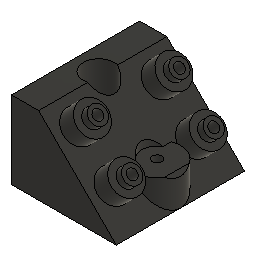
camera_block_left (Autodesk Fusion 360 design; units mm, degrees)
Autodesk Fusion 360 part; units mm, degrees
note: some values were not read from the file. Chosen so that the rebuilt part matches the saved one: which bodies a step acts on.
sketch "Skizze1" plane through (0, 0, 0) normal (0, 0, 1) x (1, 0, 0)
  line L0 (-52.0005, 0) -> (60.5, 0) construction
  line L1 (0, 48.0834) -> (0, -46.0641) construction
  line L2 (13.5, 16.5) -> (-13.5, 16.5)
  line L3 (-13.5, 16.5) -> (-13.5, -16.5)
  line L4 (-13.5, -16.5) -> (13.5, -16.5)
  line L5 (13.5, -16.5) -> (13.5, 16.5)
  line L6 (13.5, 16.5) -> (-13.5, -16.5) construction
  line L7 (-13.5, 16.5) -> (13.5, -16.5) construction
  circle A0 centre (-7.5, 0) radius 1.25
  circle A1 centre (-7.5, 0) radius 4
  circle A2 centre (7.5, 0) radius 1.25
  circle A3 centre (7.5, 0) radius 4
  circle A4 centre (7.5, 0) radius 6
  dimension "d1" = 27
  dimension "d2" = 33
  dimension "d3" = 8
  dimension "d4" = 2.5
  dimension "d5" = 8
  dimension "d6" = 2.5
  dimension "d7" = 7.5
  dimension "d8" = 7.5
  constraint horizontal L0
  constraint coincident origin L0
  constraint vertical L1
  constraint coincident origin L1
  constraint horizontal L2
  constraint perpendicular L2 L3
  constraint parallel L2 L4
  constraint parallel L3 L5
  constraint coincident L6 origin
  constraint coincident L7 origin
  constraint coincident L0 A0.centre
  constraint concentric A0 A1
  constraint coincident L0 A2.centre
  constraint concentric A2 A3
  constraint concentric A2 A4
  constraint tangent L5 A4
  measures "d1" distance of L3 L5
  measures "d2" distance of L2 L4
  measures "d3" diameter of A3
  measures "d4" diameter of A2
  measures "d5" diameter of A1
  measures "d6" diameter of A0
  measures "d7" distance of L1 A0.centre
  measures "d8" distance of origin A2.centre
extrude "Extrusion1" add sketch "Skizze1" along normal blind 28 contours A4 | L2 L3 L4 L5 | A1 | A3 makes body 1
ref_plane "Arbeitsebene1" through (0, -16.5, 0) normal (0, 1, 0) x (0, 0, 1)
sketch "Skizze2" plane through (0, -16.5, 0) normal (0, 1, 0) x (1, 0, 0)
  line L0 (-24, 0) -> (28, 0) construction
  line L1 (0, -33.563) -> (0, 23) construction
  line L2 (13.5, 0) -> (-13.5, 0)
  line L3 (-13.5, 0) -> (-13.5, -27)
  line L4 (-13.5, -27) -> (13.5, -27) construction
  line L5 (13.5, -27) -> (13.5, 0) construction
  line L6 (13.5, 0) -> (-13.5, -27)
  line L7 (-13.5, 0) -> (13.5, -27) construction
  point P0 (0, -13.5)
  dimension "d12" = 27
  dimension "d13" = 27
  constraint horizontal L0
  constraint coincident origin L0
  constraint vertical L1
  constraint coincident origin L1
  constraint horizontal L2
  constraint perpendicular L2 L3
  constraint parallel L2 L4
  constraint parallel L3 L5
  constraint coincident L6 P0
  constraint coincident L7 P0
  constraint coincident L1 P0
  constraint coincident L0 L2.start
  measures "d12" distance of L3 L5
  measures "d13" distance of L2 L4
extrude "Extrusion2" cut sketch "Skizze2" along normal blind 33 keep common part bodies 1
ref_plane "Arbeitsebene2" through (0, 0, 20) normal (0, 0, 1) x (1, 0, 0)
split "Teilen1" by plane through (0, 0, 20) normal (0, 0, 1) bodies 1 makes body 2 at (-9.3438, -11.3771, 22.8438)
delete_body "Körper entfernen1" bodies 2
ref_plane "Arbeitsebene3" through (-2.1213, 0, 11.3787) normal (0.707107, 0, 0.707107) x (0.707107, 0, -0.707107)
ref_plane "Arbeitsebene4" through (0, 0, 8.281) normal (0, 0, 1) x (1, 0, 0)
sketch "Skizze3" plane through (4.6287, 0, 4.6287) normal (0.707107, 0, 0.707107) x (0.707107, 0, -0.707107)
  line L0 (-30, 0) -> (26, 0) construction
  line L1 (-5.1652, -20) -> (-5.1652, 29) construction
  line L2 (-5.1652, 20.798) -> (-5.1652, -14.7824)
  line L3 (-0.1652, -10.5) -> (-12.6652, -10.5) construction
  line L4 (-12.6652, -10.5) -> (-12.6652, 10.5) construction
  line L5 (-12.6652, 10.5) -> (-0.1652, 10.5) construction
  line L6 (-0.1652, 10.5) -> (-0.1652, -10.5) construction
  line L7 (-0.1652, -10.5) -> (-12.6652, 10.5) construction
  line L8 (-12.6652, -10.5) -> (-0.1652, 10.5) construction
  circle A0 centre (-0.1652, 10.5) radius 1.25
  circle A1 centre (-0.1652, 10.5) radius 2.25
  circle A2 centre (-0.1652, 10.5) radius 4
  circle A3 centre (-0.1652, -10.5) radius 1.25
  circle A4 centre (-0.1652, -10.5) radius 2.25
  circle A5 centre (-0.1652, -10.5) radius 4
  circle A6 centre (-12.6652, -10.5) radius 1.25
  circle A7 centre (-12.6652, -10.5) radius 2.25
  circle A8 centre (-12.6652, -10.5) radius 4
  circle A9 centre (-12.6652, 10.5) radius 1.25
  circle A10 centre (-12.6652, 10.5) radius 2.25
  circle A11 centre (-12.6652, 10.5) radius 4
  line L9 (1.105, 8.3) -> (2.3752, 10.5)
  line L10 (2.3752, 10.5) -> (1.105, 12.7)
  line L11 (1.105, 12.7) -> (-1.4353, 12.7)
  line L12 (-1.4353, 12.7) -> (-2.7055, 10.5)
  line L13 (-2.7055, 10.5) -> (-1.4353, 8.3)
  line L14 (-1.4353, 8.3) -> (1.105, 8.3)
  line L15 (-11.395, 8.3) -> (-10.1248, 10.5)
  line L16 (-10.1248, 10.5) -> (-11.395, 12.7)
  line L17 (-11.395, 12.7) -> (-13.9353, 12.7)
  line L18 (-13.9353, 12.7) -> (-15.2055, 10.5)
  line L19 (-15.2055, 10.5) -> (-13.9353, 8.3)
  line L20 (-13.9353, 8.3) -> (-11.395, 8.3)
  line L21 (-11.395, -12.7) -> (-10.1248, -10.5)
  line L22 (-10.1248, -10.5) -> (-11.395, -8.3)
  line L23 (-11.395, -8.3) -> (-13.9353, -8.3)
  line L24 (-13.9353, -8.3) -> (-15.2055, -10.5)
  line L25 (-15.2055, -10.5) -> (-13.9353, -12.7)
  line L26 (-13.9353, -12.7) -> (-11.395, -12.7)
  line L27 (1.105, -12.7) -> (2.3752, -10.5)
  line L28 (2.3752, -10.5) -> (1.105, -8.3)
  line L29 (1.105, -8.3) -> (-1.4353, -8.3)
  line L30 (-1.4353, -8.3) -> (-2.7055, -10.5)
  line L31 (-2.7055, -10.5) -> (-1.4353, -12.7)
  line L32 (-1.4353, -12.7) -> (1.105, -12.7)
  point P0 (-6.4152, 0)
  point P1 (-0.1652, 10.5)
  point P2 (-12.6652, 10.5)
  point P3 (-12.6652, -10.5)
  point P4 (-0.1652, -10.5)
  dimension "d19" = 12.5
  dimension "d20" = 7.5
  dimension "d21" = 21
  dimension "d22" = 8
  dimension "d23" = 4.5
  dimension "d24" = 2.5
  dimension "d25" = 8
  dimension "d26" = 4.5
  dimension "d27" = 2.5
  dimension "d28" = 8
  dimension "d29" = 4.5
  dimension "d30" = 2.5
  dimension "d31" = 8
  dimension "d32" = 4.5
  dimension "d33" = 2.5
  dimension "d34" = 4.4
  dimension "d35" = 4.4
  dimension "d36" = 4.4
  dimension "d37" = 4.4
  constraint horizontal L0
  constraint coincident origin L0
  constraint vertical L1
  constraint coincident L1.start L2
  constraint horizontal L3
  constraint perpendicular L3 L4
  constraint parallel L3 L5
  constraint parallel L4 L6
  constraint coincident L7 P0
  constraint coincident L8 P0
  constraint coincident L0 P0
  constraint coincident P1 L5.end
  constraint concentric A0 A1
  constraint concentric A0 A2
  constraint coincident P4 L3.start
  constraint concentric A3 A4
  constraint concentric A4 A5
  constraint coincident P3 L3.end
  constraint concentric A6 A7
  constraint concentric A6 A8
  constraint coincident P2 L4.end
  constraint concentric A9 A10
  constraint concentric A10 A11
  constraint horizontal L32
  constraint horizontal L26
  constraint horizontal L20
  constraint horizontal L14
  measures "d19" distance of L4 L6
  measures "d20" distance of L1 L4
  measures "d21" distance of L3 L5
  measures "d22" diameter of A2
  measures "d23" diameter of A1
  measures "d24" diameter of A0
  measures "d25" diameter of A5
  measures "d26" diameter of A4
  measures "d27" diameter of A3
  measures "d28" diameter of A8
  measures "d29" diameter of A7
  measures "d30" diameter of A6
  measures "d31" diameter of A11
  measures "d32" diameter of A10
  measures "d33" diameter of A9
  measures "d34" distance of L11 L14
  measures "d35" distance of L17 L20
  measures "d36" distance of L23 L26
  measures "d37" distance of L29 L32
extrude "Extrusion3" add sketch "Skizze3" along normal blind 8 contours A1 L9 L10 | A1 L10 L11 | A1 L9 L14 | A1 L11 L12 | A1 L13 L14 | A1 L12 L13 | A2 | A4 L27 L28 | A4 L28 L29 | A4 L27 L32 | A4 L29 L30 | A4 L31 L32 | A4 L30 L31 | A5 | A7 L21 L22 | A7 L22 L23 | A7 L21 L26 | A7 L23 L24 | A7 L25 L26 | A7 L24 L25 | A8 | A10 L15 L16 | A10 L16 L17 | A10 L15 L20 | A10 L17 L18 | A10 L19 L20 | A10 L18 L19 | A11 bodies 1
extrude "Extrusion4" add sketch "Skizze3" along normal blind 10 contours A1 L9 L10 L11 L12 L13 L14 | A1 L10 | A1 L9 | A1 L11 | A1 L14 | A1 L12 | A1 L13 | A4 L27 L28 L29 L30 L31 L32 | A4 L28 | A4 L27 | A4 L29 | A4 L32 | A4 L30 | A4 L31 | A7 L21 L22 L23 L24 L25 L26 | A7 L22 | A7 L21 | A7 L23 | A7 L26 | A7 L24 | A7 L25 | A10 L15 L16 L17 L18 L19 L20 | A10 L16 | A10 L15 | A10 L17 | A10 L20 | A10 L18 | A10 L19 bodies 1
extrude "Extrusion5" cut sketch "Skizze3" along normal blind 6 contours A1 L9 L10 L11 L12 L13 L14 | A1 L9 L10 | A1 L10 L11 | A1 L9 L14 | A1 L11 L12 | A1 L13 L14 | A1 L12 L13 | A4 L27 L28 L29 L30 L31 L32 | A4 L27 L28 | A4 L28 L29 | A4 L27 L32 | A4 L29 L30 | A4 L31 L32 | A4 L30 L31 | A7 L21 L22 L23 L24 L25 L26 | A7 L21 L22 | A7 L22 L23 | A7 L21 L26 | A7 L23 L24 | A7 L25 L26 | A7 L24 L25 | A10 L15 L16 L17 L18 L19 L20 | A10 L15 L16 | A10 L16 L17 | A10 L15 L20 | A10 L17 L18 | A10 L19 L20 | A10 L18 L19 bodies 1
extrude "Extrusion6" add sketch "Skizze3" along normal blind 4.2 contours A1 L9 L10 L11 L12 L13 L14 | A1 L9 L10 | A1 L10 L11 | A1 L9 L14 | A1 L11 L12 | A1 L13 L14 | A1 L12 L13 | A4 L27 L28 L29 L30 L31 L32 | A4 L27 L28 | A4 L28 L29 | A4 L27 L32 | A4 L29 L30 | A4 L31 L32 | A4 L30 L31 | A7 L21 L22 L23 L24 L25 L26 | A7 L21 L22 | A7 L22 L23 | A7 L21 L26 | A7 L23 L24 | A7 L25 L26 | A7 L24 L25 | A10 L15 L16 L17 L18 L19 L20 | A10 L15 L16 | A10 L16 L17 | A10 L15 L20 | A10 L17 L18 | A10 L19 L20 | A10 L18 L19 bodies 1
extrude "Extrusion7" cut sketch "Skizze1" along normal blind 25 contours A1 | A3 bodies 1
extrude "Extrusion8" add sketch "Skizze1" along normal blind 8 contours A4 | A1 | A3 bodies 1
split "Teilen2" by plane through (10.2855, 0, 10.2855) normal (0.707107, 0, 0.707107) bodies 1 makes body 3 at (12.2232, -10.724, 9.2906) makes body 4 at (3.8558, -10.276, 18.6009) makes body 5 at (3.3844, 10.276, 18.1295) makes body 6 at (12.6946, 10.724, 9.762) makes body 7 at (13.4849, 0.4258, 7.6956)
delete_body "Körper entfernen2" bodies 7
combine "Kombinieren1" operation add target body 1 tool bodies 3 4 5 6
extrude "Extrusion9" cut sketch "Skizze1" along normal blind 6 contours A1 | A3 bodies 1
equation "d11 = -( 33 / 2 ) * 1 mm"
named bodies: "camera_block_left"
